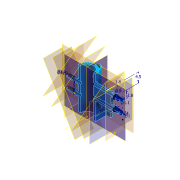
# Autodesk Inventor part: offset_cylinder
Saved by Autodesk Inventor 2021 (Build 250183000, 183)
## iProperties
Created: 2021-07-12
Part Number: offset_cylinder
Material: Generic
Document SubType Name: Modeling
Designer: Sihan
Density: 1 g/cm^3
Appearance: Default
Mass: 1.69832 g
Surface Area: 23.6767 cm^2
Volume: 1.69832 cm^3
Author: Sihan
Autodesk Inventor part; units mm, degrees
ref_plane "XZ Plane" through (0, 0, 0) normal (0, 1, 0) x (-1, 0, 0)
sketch "Sketch1" plane through (0, 0, 0) normal (0, 1, 0) x (-1, 0, 0)
  circle A0 centre (0, 0) radius 2.99
  circle A1 centre (0, 0) radius 4
  dimension "d0" = 5.98
  dimension "d1" = 8
  constraints: 2 centre point, 1 coincident
  measures "d0" diameter of A0
  measures "d1" diameter of A1
extrude "Extrusion1" add sketch "Sketch1" along normal blind 19
ref_plane "Work Plane1" through (13, 0, 0) normal (1, 0, 0) x (0, 1, 0)
sketch "Sketch2" plane through (13, 0, 0) normal (1, 0, 0) x (0, 1, 0)
  circle A0 centre (14.5, 0) radius 0.9
  circle A1 centre (9.5, 0) radius 0.9
  line L0 (19, -4) -> (19, 4) projected
  circle A2 centre (14.5, 0) radius 0.25
  circle A3 centre (9.5, 0) radius 0.25
  point P0 (0, 0)
  dimension "d5" = 1.8
  dimension "d7" = 1.8
  dimension "d9" = 4.5
  dimension "d16" = 0.5
  dimension "d18" = 0.5
  dimension "d82" = 5
  constraints: 4 centre point
  measures "d5" diameter of A0
  measures "d7" diameter of A1
  measures "d9" distance from line of L0 A0.centre
  measures "d16" diameter of A2
  measures "d18" diameter of A3
  measures "d82" distance of A1.centre A0.centre
extrude "Extrusion2" add sketch "Sketch2" against normal up to next contours A0 | A1 | A2 | A3
extrude "Extrusion3" cut sketch "Sketch2" against normal up to next contours A2 | A3
sketch "Sketch3" plane through (0, 0, 0) normal (0, 0, 1) x (1, 0, 0)
  line L0 (13, 14.75) -> (13, 14.25) projected
  line L1 (13, 14.5) -> (15.9195, 14.5)
  line L2 (13, 14.5) -> (13, 15.7)
  line L3 (13, 15.7) -> (16.5, 15.2)
  line L4 (13, 9.75) -> (13, 9.25) projected
  line L5 (13, 9.5) -> (18.6368, 9.5)
  line L6 (13, 9.5) -> (13, 10.7)
  line L7 (13, 10.7) -> (16.5, 10.2)
  line L8 (16.5, 15.2) -> (16.5, 15.05)
  line L9 (16.5, 15.05) -> (13, 15.05)
  line L10 (16.5, 10.2) -> (16.5, 10)
  line L11 (16.5, 10) -> (13, 10)
  point P0 (0, 0)
  point P1 (16.5, 7)
  dimension "d23" = 1.2
  dimension "d30" = 1.2
  dimension "d34" = 1.4
  dimension "d35" = 1.1
  dimension "d38" = 1.4
  dimension "d41" = 1
  dimension "d192" = 3.5
  dimension "d193" = 3.5
  constraints: 20 end point, 4 vertical, 3 point on line, 2 horizontal, 2 midpoint, 2 perpendicular
  measures "d23" distance of L1.start L2.end
  measures "d30" distance of L5.start L6.end
  measures "d34" diameter of L3.end L1
  measures "d35" diameter of L9 L1
  measures "d38" diameter of L7.end L5
  measures "d41" diameter of L11 L5
  measures "d192" distance of L8.end L9.end
  measures "d193" distance of L10.end L11.end
revolve "Revolution1" add sketch "Sketch3" angle 360 about axis through (13, 14.5, 0) along (1, 0, 0) separate body contours L2 L3 L8 L9
revolve "Revolution3" add sketch "Sketch3" angle 360 about axis through (13, 9.5, 0) along (1, 0, 0) separate body contours L6 L7 L10 L11
ref_plane "Work Plane2" through (0, 0, 0) normal (0.8660254, 0.5, 0) x (0, 0, 1)
ref_plane "Work Plane7" through (-6, 0, 0) normal (1, 0, 0) x (0, 1, 0)
sketch "Sketch4" plane through (-6, 0, 0) normal (1, 0, 0) x (0, 1, 0)
  circle A0 centre (12, 0) radius 0.9
  line L0 (19, -4) -> (19, 4) projected
  circle A1 centre (7, 0) radius 0.9
  line L1 (0, -4) -> (0, 4) projected
  point P0 (0, 0)
  dimension "d52" = 7
  dimension "d53" = 1.8
  dimension "d54" = 1.8
  dimension "d81" = 5
  constraints: 2 centre point
  measures "d52" distance from line of L0 A0.centre
  measures "d53" diameter of A0
  measures "d54" diameter of A1
  measures "d81" distance of A1.centre A0.centre
extrude "Extrusion4" add sketch "Sketch4" along normal up to next bodies 1
sketch "Sketch5" plane through (-6, 12, 0) normal (-1, 0, 0) x (0, 0, 1)
  circle A0 centre (0, 0) radius 0.9 projected
  circle A1 centre (0, 0) radius 0.9 projected
  circle A2 centre (0, 0) radius 0.25
  circle A3 centre (0, -5) radius 0.9 projected
  circle A4 centre (0, -5) radius 0.25
  dimension "d58" = 0.5
  dimension "d143" = 0.5
  constraints: 2 centre point, 2 coincident
  measures "d58" diameter of A2
  measures "d143" diameter of A4
extrude "Extrusion5" cut sketch "Sketch5" against normal up to next contours A2 | A4 bodies 1
sketch "Sketch6" plane through (0, 0, 0) normal (0, 0, 1) x (1, 0, 0)
  line L0 (-6, 11.1) -> (-6, 12.9) projected
  line L1 (-6, 12) -> (-10.2091, 12)
  line L2 (-6, 12) -> (-6, 13.2)
  line L3 (-6, 13.2) -> (-9.5, 12.7)
  line L4 (-9.5, 12.7) -> (-9.5, 12.55)
  line L5 (-9.5, 12.55) -> (-6, 12.55)
  line L6 (-6, 6.1) -> (-6, 7.9) projected
  line L7 (-6, 7) -> (-10.2091, 7)
  line L8 (-6, 7) -> (-6, 8.2)
  line L9 (-6, 8.2) -> (-9.5, 7.7)
  line L10 (-9.5, 7.7) -> (-9.5, 7.55)
  line L11 (-9.5, 7.55) -> (-6, 7.55)
  point P0 (0, 0)
  point P1 (-6, 6.1)
  point P2 (-6, 7.9)
  dimension "d62" = 1.1
  dimension "d63" = 1.4
  dimension "d64" = 1.2
  dimension "d108" = 5
  constraints: 20 end point, 3 vertical, 2 point on line, 1 horizontal, 1 midpoint, 1 perpendicular, 13 other
  measures "d62" diameter of L5 L1
  measures "d63" diameter of L3.end L1
  measures "d64" distance of L1.start L2.end
  measures "d108" distance of L1.start L7.start
revolve "Revolution5" add sketch "Sketch6" angle 360 about axis through (-6, 12, 0) along (-1, 0, 0) separate body contours L5 L4 L3 L2 L0
ref_plane "Work Plane8" through (0, 0, 0) normal (0.8660254, -0.5, 0) x (0, 0, 1)
ref_plane "Work Plane9" through (-9.1799, 5.3, 0) normal (0.8660254, -0.5, 0) x (0, 0, 1)
ref_plane "Work Plane10" through (-13.077, 7.55, 0) normal (0.8660254, -0.5, 0) x (0, 0, 1)
ref_plane "Work Plane14" through (-4.3301, -2.5, 0) normal (0.8660254, 0.5, 0) x (0, 0, 1)
split "Split7" plane through (-4.3301, -2.5, 0) removes the side toward (-0.8660254, -0.5, 0) bodies 4
pattern_of_nothing "Mirror1"
pattern_of_nothing "Mirror2"
revolve "Revolution9" add sketch "Sketch6" angle 360 about axis through (-6, 7, 0) along (-1, 0, 0) separate body contours L11 L10 L9 L8 L6
ref_plane "Work Plane17" through (0, 0, -5) normal (0, 0, 1) x (1, 0, 0)
sketch "Sketch12" plane through (0, 0, -5) normal (0, 0, 1) x (1, 0, 0)
  line L0 (0, 4.5) -> (0, 4.5) construction
  line L1 (0, 4) -> (0, 4)
  line L2 (0, 5) -> (0, 5)
  arc A0 (0, 4) -> (0, 5) centre (0, 4.5) ccw
  arc A1 (0, 5) -> (0, 4) centre (0, 4.5) ccw
  line L3 (0, 14.5) -> (0, 14.5) construction
  line L4 (0, 14) -> (0, 14)
  line L5 (0, 15) -> (0, 15)
  arc A2 (0, 14) -> (0, 15) centre (0, 14.5) ccw
  arc A3 (0, 15) -> (0, 14) centre (0, 14.5) ccw
  line L6 (4, 0) -> (-4, 0) projected
  line L7 (4, 19) -> (-4, 19) projected
  point P0 (0, 0)
  point P1 (0, 4.5)
  point P2 (0, 0)
  dimension "d118" = 0.5
  dimension "d121" = 0
  dimension "d122" = 0
  dimension "d123" = 0.5
  dimension "d190" = 4.5
  dimension "d191" = 10
  constraints: 16 end point, 8 point on circle, 8 tangent, 4 centre point, 3 midpoint, 2 horizontal, 2 parallel, 2 vertical alignment
  measures "d118" radius of A1
  measures "d121" distance of L0.start L0.end
  measures "d122" distance of L3.start L3.end
  measures "d123" radius of A3
  measures "d190" distance from line of L7 point (0, 14.5)
  measures "d191" distance of point (0, 4.5) point (0, 14.5)
extrude "Extrusion9" cut sketch "Sketch12" along normal up to next bodies 1
ref_plane "Work Plane18" through (0, 3, 0) normal (0, -1, 0) x (1, 0, 0)
sketch "Sketch13" plane through (0, 3, 0) normal (0, -1, 0) x (1, 0, 0)
  circle A0 centre (0, 0) radius 4 projected
  circle A1 centre (0, -4) radius 1.5
  circle A2 centre (0, -4) radius 2
  point P0 (-1.9365, -3.5)
  point P1 (1.9365, -3.5)
  point P2 (1.4734, -3.7188)
  point P3 (-1.4734, -3.7187)
  dimension "d194" = 3
  dimension "d195" = 0.5
  constraints: 2 centre point, 2 other
  measures "d194" diameter of A1
  measures "d195" radial gap between concentric circles of A2 A1
extrude "Extrusion10" add sketch "Sketch13" against normal blind 13 contours A0 A1 A2 picked at (1.7998, -4.2779) bodies 1
pattern_of_nothing "Mirror3"
sketch "Sketch20" plane through (0, 0, 0) normal (0, -1, 0) x (1, 0, 0)
  line L0 (-4, -9) -> (4, -9)
  line L1 (4, -9) -> (4, 9)
  line L2 (4, 9) -> (-4, 9)
  line L3 (-4, 9) -> (-4, -9)
  line L4 (-4, -9) -> (4, 9) construction
  line L5 (4, -9) -> (-4, 9) construction
  circle A0 centre (0, 0) radius 4 projected
  point P0 (-4, 0)
  point P1 (4, 0)
  dimension "d161" = 8
  dimension "d162" = 18
  constraints: 12 end point, 2 midpoint, 2 parallel, 1 horizontal, 1 perpendicular
  measures "d161" distance of L1.end L2.end
  measures "d162" distance of L0.end L1.end
extrude "Extrusion16" add sketch "Sketch20" against normal blind 2 contours L3 A0 L1 L0 | L3 L2 L1 A0 bodies 1
sketch "Sketch21" plane through (4, 0, 9) normal (1, 0, 0) x (0, 0, -1)
  line L0 (9, 2) -> (0, 2) projected
  line L1 (18, 0) -> (0, 0) projected
  line L2 (0, 2) -> (1, 2)
  line L3 (1, 2) -> (1, 0)
  line L4 (1, 0) -> (0, 0)
  line L5 (0, 0) -> (0, 2)
  line L6 (3, 0) -> (4, 0)
  line L7 (4, 0) -> (4, 2)
  line L8 (4, 2) -> (3, 2)
  line L9 (3, 2) -> (3, 0)
  point P0 (9, 0)
  point P1 (4, 0)
  point P2 (1, 2)
  dimension "d165" = 1
  dimension "d166" = 2
  dimension "d167" = 1
  constraints: 16 end point, 4 parallel, 3 point on line, 2 horizontal, 2 perpendicular
  measures "d165" distance between parallel lines of L3 L5
  measures "d166" distance between parallel lines of L9 L3
  measures "d167" distance between parallel lines of L9 L7
extrude "Extrusion17" add sketch "Sketch21" along normal blind 2 contours L7 L1 L9 L0 | L3 L1 L5 L0 bodies 1
mirror "Mirror4" about plane through (0, 0, 0) normal (0, 0, 1) of "Extrusion17" bodies 1
mirror "Mirror5" about plane through (0, 0, 0) normal (1, 0, 0) of "Extrusion17", "Mirror4" bodies 1
sketch "Sketch22" plane through (0, 3, 0) normal (0, -1, 0) x (1, 0, 0)
  circle A0 centre (0, 0) radius 2.99 projected
  arc A1 (-1.9365, -3.5) -> (1.9365, -3.5) centre (0, -4) ccw projected
  arc A2 (-1.9365, -3.5) -> (-1.4734, -3.7187) centre (0, 0) ccw projected
  arc A3 (-1.4734, -3.7187) -> (1.4734, -3.7188) centre (0, 0) ccw projected
  arc A4 (-1.4734, -3.7187) -> (1.4734, -3.7188) centre (0, -4) ccw projected
  arc A5 (1.4734, -3.7188) -> (1.9365, -3.5) centre (0, 0) ccw projected
  arc A6 (1.9365, -3.5) -> (-1.9365, -3.5) centre (0, 0) ccw projected
extrude "Extrusion18" add sketch "Sketch22" along normal blind 1 contours A2 A4 A5 A1 | A3 A4 bodies 1
sketch "Sketch23" plane through (0, 16, 0) normal (0, 1, 0) x (1, 0, 0)
  circle A0 centre (0, 0) radius 2.99 projected
  arc A1 (1.9365, 3.5) -> (-1.9365, 3.5) centre (0, 4) ccw projected
  arc A2 (1.9365, 3.5) -> (1.4734, 3.7188) centre (0, 0) ccw projected
  arc A3 (1.4734, 3.7188) -> (-1.4734, 3.7187) centre (0, 0) ccw projected
  arc A4 (1.4734, 3.7188) -> (-1.4734, 3.7187) centre (0, 4) ccw projected
  arc A5 (-1.4734, 3.7187) -> (-1.9365, 3.5) centre (0, 0) ccw projected
  arc A6 (-1.9365, 3.5) -> (1.9365, 3.5) centre (0, 0) ccw projected
extrude "Extrusion19" add sketch "Sketch23" along normal blind 2 contours A2 A4 A5 A1 bodies 1
ref_plane "Work Plane23" through (11, 0, 0) normal (-1, 0, 0) x (0, 1, 0)
ref_plane "Work Plane12" through (0, 0, 0) normal (-1, 0, 0) x (0, 1, 0)
sketch "Sketch24" plane through (11, 0, 0) normal (-1, 0, 0) x (0, 1, 0)
  circle A0 centre (14.5, 0) radius 1.2 projected
  circle A1 centre (9.5, 0) radius 0.25 projected
  line L0 (14.5, 0) -> (9.5, 0) construction
  line L1 (14.5, 1.3) -> (9.5, 1.3)
  line L2 (9.5, -1.3) -> (14.5, -1.3)
  arc A2 (14.5, -1.3) -> (14.5, 1.3) centre (14.5, 0) ccw
  arc A3 (9.5, 1.3) -> (9.5, -1.3) centre (9.5, 0) ccw
  circle A4 centre (9.5, 0) radius 0.25 projected
  circle A5 centre (14.5, 0) radius 0.25 projected
  circle A6 centre (9.5, 0) radius 0.9 projected
  circle A7 centre (14.5, 0) radius 0.9 projected
  point P0 (0, 0)
  point P1 (12, 0)
  dimension "d175" = 1.3
  constraints: 8 end point, 4 point on circle, 4 tangent, 2 centre point, 1 horizontal, 1 midpoint, 1 parallel
  measures "d175" radius of A2
extrude "Extrusion20" add sketch "Sketch24" along normal up to next contours A0 | A2 L2 A3 L1 bodies 1
fillet "Fillet5" radius 0.5 2 edges at (11, 13.6, 0) (11, 8.6, 0)
fillet "Fillet6" radius 0.5 4 edges at (-3.8974, 11.9999, -0.9) (-3.8974, 12, 0.9) (-3.8974, 6.9999, -0.9) (-3.8974, 7, 0.9)
sketch "Sketch25" plane through (13, 14.5, 0) normal (1, 0, 0) x (0, 0, -1)
  circle A0 centre (0, -5) radius 0.9 projected
  circle A1 centre (0, 0) radius 0.9 projected
  circle A2 centre (0, -5) radius 0.25 projected
  circle A3 centre (0, 0) radius 0.25 projected
  circle A4 centre (0, 0) radius 0.55 projected
  circle A5 centre (0, 0) radius 1.2 projected
  circle A6 centre (0, -5) radius 0.5 projected
  circle A7 centre (0, -5) radius 1.2 projected
  point P0 (0, -14.5)
extrude "Extrusion21" cut sketch "Sketch25" against normal up to surface contours A2 | A3 | A4 | A6 round surface about axis through (0, 0, 0) along (0, 1, 0) radius 2.99 far side no bodies 1
sketch "Sketch26" plane through (-6, 12, 0) normal (-1, 0, 0) x (0, 0, 1)
  circle A0 centre (0, -5) radius 0.9 projected
  circle A1 centre (0, 0) radius 0.9 projected
  line L0 (-9, -10) -> (-8, -10) projected
  line L1 (-8, -10) -> (-8, -12) projected
  line L2 (-8, -12) -> (-9, -12) projected
  line L3 (-9, -12) -> (-9, -10) projected
  line L4 (-6, -10) -> (-5, -10) projected
  line L5 (-5, -10) -> (-5, -12) projected
  line L6 (-5, -12) -> (-6, -12) projected
  line L7 (-6, -12) -> (-6, -10) projected
  line L8 (5, -12) -> (5, -10) projected
  line L9 (5, -10) -> (6, -10) projected
  line L10 (6, -10) -> (6, -12) projected
  line L11 (6, -12) -> (5, -12) projected
  line L12 (9, -10) -> (9, -12) projected
  line L13 (9, -12) -> (8, -12) projected
  line L14 (8, -12) -> (8, -10) projected
  line L15 (8, -10) -> (9, -10) projected
  circle A2 centre (0, 0) radius 0.25 projected
  circle A3 centre (0, -5) radius 0.25 projected
  circle A4 centre (0, 0) radius 1.2 projected
  circle A5 centre (0, 0) radius 0.55 projected
  circle A6 centre (0, -5) radius 1.2 projected
  circle A7 centre (0, -5) radius 0.55 projected
  point P0 (0, -12)
extrude "Extrusion22" cut sketch "Sketch26" against normal up to surface contours A5 round surface about axis through (0, 0, 0) along (0, 1, 0) radius 2.99 far side no bodies 1
sketch "Sketch27" plane through (-6, 7, 0) normal (-1, 0, 0) x (0, 0, 1)
  circle A0 centre (0, 5) radius 0.55 projected
  circle A1 centre (0, 0) radius 0.9 projected
  circle A2 centre (0, 5) radius 0.9 projected
  line L0 (-9, -5) -> (-8, -5) projected
  line L1 (-8, -5) -> (-8, -7) projected
  line L2 (-8, -7) -> (-9, -7) projected
  line L3 (-9, -7) -> (-9, -5) projected
  line L4 (-6, -5) -> (-5, -5) projected
  line L5 (-5, -5) -> (-5, -7) projected
  line L6 (-5, -7) -> (-6, -7) projected
  line L7 (-6, -7) -> (-6, -5) projected
  line L8 (5, -7) -> (5, -5) projected
  line L9 (5, -5) -> (6, -5) projected
  line L10 (6, -5) -> (6, -7) projected
  line L11 (6, -7) -> (5, -7) projected
  line L12 (9, -5) -> (9, -7) projected
  line L13 (9, -7) -> (8, -7) projected
  line L14 (8, -7) -> (8, -5) projected
  line L15 (8, -5) -> (9, -5) projected
  circle A3 centre (0, 0) radius 0.25 projected
  circle A4 centre (0, 5) radius 1.2 projected
  circle A5 centre (0, 5) radius 0.55 projected
  circle A6 centre (0, 0) radius 1.2 projected
  circle A7 centre (0, 0) radius 0.55 projected
  point P0 (0, -7)
extrude "Extrusion23" cut sketch "Sketch27" against normal up to surface contours A7 round surface about axis through (0, 0, 0) along (0, 1, 0) radius 2.99 far side no bodies 1
combine bodies "Combine1" operation type add bodies to combine 1 2 3 4 5
split "Split10" plane through (0, 0, 0) removes the side toward (0, 0, 1) bodies 1
ref_plane "Work Plane11" through (0, 0, 0) normal (1, 0, 0) x (0, 1, 0)
ref_plane "Work Plane13" through (0, 0, 0) normal (-1, 0, 0) x (0, 1, 0)
ref_plane "Work Plane19" through (0, 0, 0) normal (1, 0, 0) x (0, 1, 0)
ref_plane "Work Plane20" through (0, 0, 0) normal (0, 0, 1) x (1, 0, 0)
ref_plane "Work Plane21" through (0, 0, 0) normal (0, 0, -1) x (-1, 0, 0)
ref_plane "Work Plane22" through (0, 0, 0) normal (0, 0, -1) x (-1, 0, 0)
body "Solid1"
